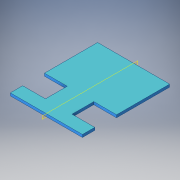
# Autodesk Inventor part: RhinoBottomFloorPlate04
Saved by Autodesk Inventor 2016 SP1 (Build 200210100, 210)
## iProperties
Created: 2015-12-30
Part Number: RhinoBottomFloorPlate04
Material: Wood (Birch)
Document SubType Name: Modeling
Designer: steele
Density: 0.55 g/cm^3
Appearance: Cyan
Mass: 2212.89 g
Surface Area: 5006.76 cm^2
Volume: 4023.43 cm^3
Author: steele
Autodesk Inventor part; units mm, degrees
ref_plane "XZ Plane" through (0, 0, 0) normal (0, 1, 0) x (-1, 0, 0)
ref_plane "XY Plane" through (0, 0, 0) normal (0, 0, 1) x (1, 0, 0)
sketch "Sketch1" plane through (0, 0, 0) normal (0, 1, 0) x (-1, 0, 0)
  line L0 (-241.3, 292.1) -> (-241.3, -292.1)
  line L1 (-241.3, -292.1) -> (241.3, -292.1)
  line L2 (241.3, -292.1) -> (241.3, 292.1)
  line L3 (241.3, 292.1) -> (-241.3, 292.1)
  line L4 (-241.3, 292.1) -> (241.3, -292.1) construction
  line L5 (-241.3, -292.1) -> (241.3, 292.1) construction
  point P0 (0, 0)
  dimension "baseLength" = 584.2
  dimension "baseWidth" = 482.6
  constraints: 12 end point, 2 midpoint, 2 parallel, 1 perpendicular, 1 vertical
  measures "baseLength" distance of L0.start L0.end
  measures "baseWidth" distance of L2.end L0.start
extrude "Extrusion1" add sketch "Sketch1" along normal blind 17.78
sketch "Sketch2" plane through (0, 0, 0) normal (0, -1, 0) x (1, 0, 0)
  line L0 (241.3, 292.1) -> (241.3, -292.1) projected
  line L1 (241.3, 209.55) -> (88.9, 209.55)
  line L2 (88.9, 209.55) -> (88.9, 63.5)
  line L3 (88.9, 63.5) -> (241.3, 63.5)
  line L4 (241.3, 63.5) -> (241.3, 209.55)
  line L5 (-241.3, 292.1) -> (241.3, 292.1) projected
  point P0 (0, 0)
  dimension "backToEndOfGearBox" = 82.55
  dimension "backToFrontOfGearBox" = 228.6
  dimension "wdithForGearBox" = 152.4
  constraints: 8 end point, 2 perpendicular, 2 point on line, 1 collinear, 1 horizontal
  measures "backToEndOfGearBox" distance between parallel lines of L1 L5
  measures "backToFrontOfGearBox" distance between parallel lines of L3 L5
  measures "wdithForGearBox" distance between parallel lines of L2 L0
extrude "Extrusion2" cut sketch "Sketch2" against normal through all
mirror "Mirror1" about plane through (0, 0, 0) normal (1, 0, 0) of "Extrusion2"
equation "\"spaceingAlongSides\" = 3.175"
equation "\"distanceFromBackForEndBolt\" = 38.1"
equation "\"spacingForBolt\" = 25.4"
equation "\"widthOfSpacingForBolt\" = 12.7"
equation "\"lengthOfSpacingForBolt\" = 25.4"
body "Solid1"
